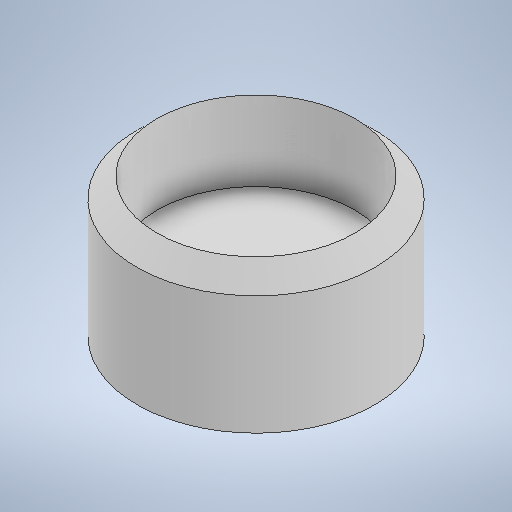
# Autodesk Inventor part: base_1.0
Saved by Autodesk Inventor 2025.1 (Build 291241000, 241)
## iProperties
Created: 2025-03-17
Part Number: base_1.0
Material: Generic
Document SubType Name: Modeling
Designer: jdoct
Density: 1 g/cm^3
Appearance: Default
Author: jdoct
Autodesk Inventor part; units mm, degrees
ref_plane "YZ Plane" through (0, 0, 0) normal (1, 0, 0) x (0, 1, 0)
ref_plane "XZ Plane" through (0, 0, 0) normal (0, 1, 0) x (-1, 0, 0)
ref_plane "XY Plane" through (0, 0, 0) normal (0, 0, 1) x (1, 0, 0)
sketch "Sketch2" plane through (0, 0, 0) normal (0, 0, 1) x (1, 0, 0)
  line L0 (0, 0) -> (19.05, 0)
  line L1 (19.05, 0) -> (19.05, 19.05)
  line L2 (19.05, 19.05) -> (15.875, 19.05) construction
  line L3 (15.875, 19.05) -> (15.875, 22.225) construction
  line L4 (15.875, 22.225) -> (19.05, 19.05)
  line L5 (15.875, 22.225) -> (0, 22.225)
  line L6 (0, 22.225) -> (0, 0)
  dimension "d3" = 19.05
  dimension "d4" = 19.05
  dimension "d10" = 3.175
  dimension "d11" = 3.175
  constraints: 14 end point, 3 horizontal, 3 perpendicular
  measures "d3" distance of L0.start L0.end
  measures "d4" distance of L0.end L1.end
  measures "d10" distance of L1.end L2.end
  measures "d11" distance of L2.end L3.end
revolve "Revolution2" add sketch "Sketch2" angle 360 about axis through (0, 22.225, 0) along (0, -1, 0)
sketch "Sketch4" plane through (0, 22.225, 0) normal (0, 1, 0) x (1, 0, 0)
  circle A0 centre (0, 0) radius 15.875 projected
extrude "Extrusion3" cut sketch "Sketch4" against normal blind 12.7
body "Solid3"
